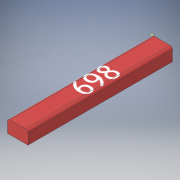
# Autodesk Inventor part: Bumper Long
Saved by Autodesk Inventor 2018.2 (Build 222227000, 227)
## iProperties
Created: 2018-01-13
Part Number: Bumper Long
Material: Generic
Document SubType Name: Modeling
Designer: jahu2
Density: 1 g/cm^3
Appearance: Default
Author: jahu2
Autodesk Inventor part; units mm, degrees
ref_plane "YZ Plane" through (0, 0, 0) normal (1, 0, 0) x (0, 1, 0)
ref_plane "XZ Plane" through (0, 0, 0) normal (0, 1, 0) x (-1, 0, 0)
ref_plane "XY Plane" through (0, 0, 0) normal (0, 0, 1) x (1, 0, 0)
sketch "Sketch1" plane through (0, 0, 0) normal (0, 0, 1) x (1, 0, 0)
  line L0 (0, 0) -> (101.6, 0)
  line L1 (101.6, 0) -> (101.6, -63.5)
  line L2 (101.6, -63.5) -> (0, -63.5)
  line L3 (0, -63.5) -> (0, 0)
  dimension "d0" = 101.6
  dimension "d1" = 63.5
  constraints: 8 end point, 2 parallel, 1 horizontal, 1 perpendicular
  measures "d0" distance of L1.end L2.end
  measures "d1" distance of L0.end L1.end
extrude "Extrusion1" add sketch "Sketch1" along normal blind 711.2
fillet "Fillet1" radius 12.7 2 edges at (101.6, 0, 355.6) (0, 0, 355.6)
sketch "Sketch2" plane through (12.7, 0, 0) normal (0, 1, 0) x (1, 0, 0)
  line L0 (-6.4537, -428.3305) -> (-6.4537, -369.6841) construction
  line L1 (-6.4537, -369.6841) -> (304.8235, -369.6841) construction
  line L2 (304.8235, -369.6841) -> (304.8235, -428.3305) construction
  line L3 (304.8235, -428.3305) -> (-6.4537, -428.3305) construction
  point P0 (-12.7, 0)
  constraints: 2 other
body "Solid1"
